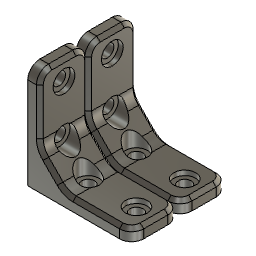
_vertical to vertical v2.d84c17af-223a-4e26-a2c8-23d5d27c0e32 (Autodesk Fusion 360 design; units mm, degrees)
Autodesk Fusion 360 part; units mm, degrees
sketch "Sketch1" plane through (0, 0, 0) normal (1, 0, 0) x (0, 1, 0)
  line L0 (0, 0) -> (0, 100) construction
  line L1 (10, 0) -> (-10, 0) construction
  line L2 (-10, 0) -> (-10, 100) construction
  line L3 (-10, 100) -> (10, 100) construction
  line L4 (10, 100) -> (10, 0) construction
  line L5 (10, 0) -> (-10, 100) construction
  line L6 (-10, 0) -> (10, 100) construction
  circle A0 centre (0, 15) radius 2.65
  circle A1 centre (0, 35) radius 2.65
  point P0 (0, 50)
  dimension "d1" = 100
  dimension "d2" = 20
  dimension "d3" = 5.3
  dimension "d4" = 15
  dimension "d5" = 5.3
  dimension "d6" = 20
  constraint coincident L0.start origin
  constraint vertical L0
  constraint horizontal L1
  constraint perpendicular L1 L2
  constraint parallel L1 L3
  constraint parallel L2 L4
  constraint coincident L5 P0
  constraint coincident L6 P0
  constraint midpoint L0 P0
  constraint coincident L0 A0.centre
  constraint coincident L0 A1.centre
  measures "d1" distance of L0.start L0.end
  measures "d2" distance of L2.end L3.end
  measures "d3" diameter of A0
  measures "d4" distance of L0.start A0.centre
  measures "d5" diameter of A1
  measures "d6" distance of A0.centre A1.centre
sketch "Sketch2" plane through (0, 0, 0) normal (0, 0, 1) x (1, 0, 0)
  line L0 (0, 0) -> (57.6272, 0) construction
  circle A0 centre (15, 0) radius 2.65 construction
  circle A1 centre (35, 0) radius 2.65 construction
  dimension "d7" = 5.3
  dimension "d8" = 5.3
  dimension "d9" = 15
  dimension "d10" = 20
  constraint coincident L0.start origin
  constraint horizontal L0
  constraint coincident L0 A0.centre
  constraint coincident L0 A1.centre
  measures "d7" diameter of A0
  measures "d8" diameter of A1
  measures "d9" distance of A0.centre L0.start
  measures "d10" distance of A0.centre A1.centre
sketch "Sketch3" plane through (0, 0, 0) normal (0, 1, 0) x (1, 0, 0)
  line L0 (0, 0) -> (0, -35)
  line L1 (0, -35) -> (0, -43)
  line L2 (0, 0) -> (35, 0)
  line L3 (35, 0) -> (43, 0)
  line L4 (0, -43) -> (5, -43)
  line L5 (43, 0) -> (43, -5)
  line L6 (43, -5) -> (5, -5)
  line L7 (5, -5) -> (5, -43)
  point P0 (0, -35)
  point P1 (0, -15)
  point P2 (35, 0)
  point P3 (15, 0)
  dimension "d11" = 8
  dimension "d12" = 8
  dimension "d13" = 5
  dimension "d14" = 5
  constraint coincident L0.start L2.start
  constraint coincident P0 L0.end
  constraint parallel L0 L1
  constraint coincident P2 L2.end
  constraint perpendicular L0 L3
  constraint perpendicular L1 L4
  constraint perpendicular L3 L5
  constraint perpendicular L0 L6
  constraint perpendicular L4 L7
  measures "d11" distance of P0 L1.end
  measures "d12" distance of P2 L3.end
  measures "d13" distance of L1.end L4.end
  measures "d14" distance of L3.end L5.end
extrude "Extrude1" add sketch "Sketch3" along normal mid plane 20 makes body 1
ref_plane "WorkPlane1" through (21.5, 0, 3) normal (0, 0, -1) x (-1, 0, 0)
ref_plane "WorkPlane2" through (3, 0, 21.5) normal (-1, 0, 0) x (0, 0, 1)
sketch "Sketch4" plane through (0, 0, 3) normal (0, 0, -1) x (-1, 0, 0)
  circle A0 centre (-35, 0) radius 2.65
  circle A1 centre (-15, 0) radius 2.65
  circle A2 centre (-35, 0) radius 4.5
  circle A3 centre (-15, 0) radius 4.5
  point P0 (-35, 0)
  point P1 (-15, 0)
  dimension "d19" = 9
  dimension "d20" = 9
  constraint concentric A0 A2
  constraint coincident P1 A1.centre
  measures "d19" diameter of A2
  measures "d20" diameter of A3
extrude "Extrude2" cut sketch "Sketch4" against normal blind 2 contours A0 | A1 | A2 | A3 bodies 1
extrude "Extrude3" cut sketch "Sketch4" along normal blind 3 contours A0 | A1 bodies 1
sketch "Sketch5" plane through (3, 0, 0) normal (-1, 0, 0) x (0, -1, 0)
  circle A0 centre (0, 15) radius 2.65
  circle A1 centre (0, 35) radius 2.65
  circle A2 centre (0, 35) radius 4.5
  circle A3 centre (0, 15) radius 4.5
  dimension "d25" = 9
  dimension "d26" = 9
  constraint concentric A1 A2
  constraint concentric A0 A3
  measures "d25" diameter of A2
  measures "d26" diameter of A3
extrude "Extrude4" cut sketch "Sketch5" against normal blind 2 contours A0 | A1 | A2 | A3 bodies 1
extrude "Extrude5" cut sketch "Sketch5" along normal blind 3 contours A0 | A1 bodies 1
fillet "Fillet2" radius 5 4 edges at (43, -10, 2.5) (43, 10, 2.5) (2.5, -10, 43) (2.5, 10, 43) on bodies 1
chamfer "Chamfer1" distance 10.467 angle 45 1 edges at (5, 0, 5) on bodies 1
fillet "Fillet1" radius 7.684 4 edges at (15.467, 7.2379, 5) (15.467, -7.2379, 5) (5, -7.2379, 15.467) (5, 7.2379, 15.467) on bodies 1
chamfer "Chamfer2" distance 1.427 angle 45 12 edges at (10.2335, -10, 10.2335) (15.7093, -10, 5.5849) (28.3249, -10, 5) (5, -10, 28.3249) (5.5849, -10, 15.7093) (28.3249, 10, 5) (5, 10, 28.3249) (5.5849, 10, 15.7093) (10.2335, 10, 10.2335) (15.7093, 10, 5.5849) (43, 0, 5) (5, 0, 43) on bodies 1
copy_body "CopyPasteBodies1" bodies 1 makes body 2
move_body "Move1" bodies 2 to x (1, 0, 0) y (0, 1, 0) z (0, 0, 1) at (0, 20, 0)
combine "Combine1" operation add target body 2 tool bodies 1
